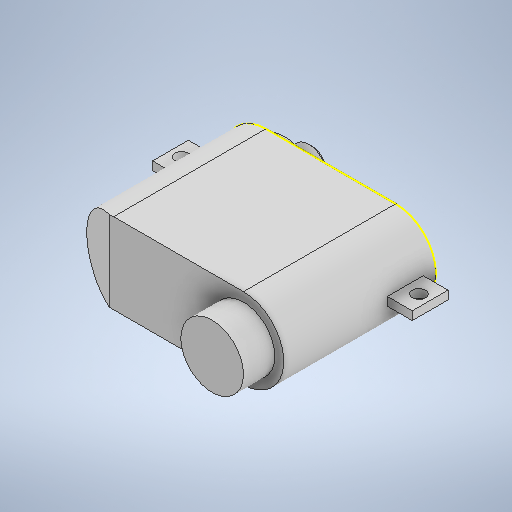
# Autodesk Inventor part: OCS-D008 B
Saved by Autodesk Inventor 2025 (Build 290162000, 162)
## iProperties
Created: 2024-09-10
Part Number: OCS-D008 B
Material: Типовые
Document SubType Name: Modeling
Designer: Andrey
Density: 1 g/cm^3
Appearance: По умолчанию
Author: Andrey
Autodesk Inventor part; units mm, degrees
ref_plane "YZ Plane" through (0, 0, 0) normal (1, 0, 0) x (0, 1, 0)
ref_plane "XZ Plane" through (0, 0, 0) normal (0, 1, 0) x (-1, 0, 0)
ref_plane "XY Plane" through (0, 0, 0) normal (0, 0, 1) x (1, 0, 0)
sketch "Эскиз1" plane through (0, 0, 0) normal (0, 0, 1) x (1, 0, 0)
  line L0 (-11.75, -4.5) -> (11.75, -4.5)
  line L1 (11.75, -4.5) -> (11.75, 4.5)
  line L2 (11.75, 4.5) -> (-11.75, 4.5)
  line L3 (-11.75, 4.5) -> (-11.75, -4.5)
  line L4 (-11.75, -4.5) -> (11.75, 4.5) construction
  line L5 (11.75, -4.5) -> (-11.75, 4.5) construction
  point P0 (0, 0)
  dimension "d0" = 23.5
  dimension "d1" = 9
  constraints: 12 end point, 2 midpoint, 2 parallel, 1 horizontal, 1 perpendicular
  measures "d0" distance of L2.end L1.end
  measures "d1" distance of L1.end L0.end
extrude "Выдавливание1" add sketch "Эскиз1" along normal mid plane 17
sketch "Эскиз2" plane through (0, 0, 0) normal (0, 1, 0) x (-1, 0, 0)
  line L0 (14.5, -3.1) -> (-14.5, -3.1)
  line L1 (-14.5, -3.1) -> (-14.5, -7.1)
  line L2 (-14.5, -7.1) -> (14.5, -7.1)
  line L3 (14.5, -7.1) -> (14.5, -3.1)
  line L4 (-11.75, 8.5) -> (11.75, 8.5) projected
  line L5 (0, 8.5) -> (0, -8.5)
  line L6 (11.75, -8.5) -> (-11.75, -8.5) projected
  line L7 (14.5, -5.1) -> (-14.5, -5.1)
  line L8 (13.25, -5.1) -> (-13.25, -5.1)
  circle A0 centre (13.25, -5.1) radius 0.75
  circle A1 centre (-13.25, -5.1) radius 0.75
  point P0 (0, 0)
  point P1 (0, -7.1)
  point P2 (0, -5.1)
  dimension "d4" = 29
  dimension "d5" = 4
  dimension "d6" = 26.5
  dimension "d7" = 1.5
  dimension "d8" = 1.5
  dimension "d9" = 3.4
  constraints: 14 end point, 7 midpoint, 3 point on line, 2 centre point, 2 coincident, 2 parallel, 1 horizontal, 1 perpendicular
  measures "d4" distance of L2.end L1.end
  measures "d5" distance of L1.end L0.end
  measures "d6" distance of L8.start L8.end
  measures "d7" diameter of A0
  measures "d8" diameter of A1
  measures "d9" distance between parallel lines of L6 L8
extrude "Выдавливание2" add sketch "Эскиз2" along normal mid plane 0.95 contours L3 L7 A0 L5 L0 | L5 L7 A1 L1 L0 | L3 L2 L5 L7 A0 | L5 L2 L1 L7 A1
fillet "Сопряжение1" radius 4.5 4 edges at (-11.75, -4.5, 0) (-11.75, 4.5, 0) (11.75, 4.5, 0) (11.75, -4.5, 0)
sketch "Эскиз3" plane through (0, 0, 8.5) normal (0, 0, 1) x (1, 0, 0)
  arc A0 (7.25, -4.5) -> (7.25, 4.5) centre (7.25, 0) ccw projected
  circle A1 centre (7.25, 0) radius 3.5
  point P0 (0, 0)
  dimension "d13" = 7
  constraints: 1 centre point, 1 coincident
  measures "d13" diameter of A1
extrude "Выдавливание3" add sketch "Эскиз3" along normal blind 3.5
sketch "Эскиз4" plane through (-7.25, 4.5, -8.5) normal (0, 1, 0) x (1, 0, 0)
  line L0 (0, -17) -> (-4.5, -17) projected
  line L1 (-4.5, -17) -> (-4.5, -15.5)
  line L2 (-4.5, 0) -> (-4.5, -17) projected
  line L3 (-4.5, -17) -> (-0.5, -17)
  line L4 (-0.5, -17) -> (-4.5, -15.5)
  point P0 (7.25, -8.5)
  dimension "d16" = 1.5
  dimension "d17" = 4
  constraints: 6 end point, 2 point on line
  measures "d16" distance of L0.end L1.end
  measures "d17" distance of L2.end L3.end
extrude "Выдавливание4" cut sketch "Эскиз4" against normal blind 20
sketch "Эскиз5" plane through (0, 0, -8.5) normal (0, 0, -1) x (-1, 0, 0)
  line L0 (14.5, -0.475) -> (14.5, 0.475) projected
  line L1 (14.5, 0) -> (-14.5, 0)
  line L2 (-14.5, -0.475) -> (-14.5, 0.475) projected
  circle A0 centre (5.95, 0) radius 4
  line L3 (12.5, 0.475) -> (12.5, -0.475) projected
  line L4 (12.5, 0) -> (14, 0)
  line L5 (14, 0.475) -> (14, -0.475) projected
  line L6 (13.25, 0) -> (5.95, 0)
  point P0 (0, 0)
  dimension "d20" = 8
  dimension "d21" = 7.3
  constraints: 6 end point, 5 midpoint, 1 centre point, 1 point on line
  measures "d20" diameter of A0
  measures "d21" distance of L6.start L6.end
extrude "Выдавливание5" add sketch "Эскиз5" along normal blind 0.8
sketch "Эскиз6" plane through (-5.95, 0, -9.3) normal (0, 0, -1) x (-1, 0, 0)
  circle A0 centre (0, 0) radius 1.925
  point P0 (-5.95, 0)
  dimension "d24" = 3.85
  constraints: 1 centre point
  measures "d24" diameter of A0
extrude "Выдавливание6" add sketch "Эскиз6" along normal blind 3
chamfer "Фаска1" distance 0.3 angle 45 1 edges at (-4.025, 0, -12.3)
sketch "Эскиз7" plane through (0, 0, -8.5) normal (0, 0, -1) x (-1, 0, 0)
  circle A0 centre (5.95, 0) radius 4 projected
  arc A1 (-7.25, 4.5) -> (-7.25, -4.5) centre (-7.25, 0) ccw projected
  line L0 (-7.25, -4.5) -> (7.25, -4.5) projected
  arc A2 (7.25, -4.5) -> (7.25, 4.5) centre (7.25, 0) ccw projected
  line L1 (7.25, 4.5) -> (-7.25, 4.5) projected
  line L2 (7.25, -4.5) -> (-7.25, -4.5)
  line L3 (-7.25, -4.5) -> (-7.25, 4.5)
  line L4 (-7.25, 4.5) -> (7.25, 4.5)
  line L5 (7.25, 4.5) -> (7.25, -4.5)
  circle A3 centre (5.95, 0) radius 1.925 projected
  circle A4 centre (5.95, 0) radius 4 projected
  circle A5 centre (5.95, 0) radius 1.625 projected
  point P0 (0, 0)
  constraints: 8 end point, 2 parallel, 1 horizontal, 1 perpendicular
